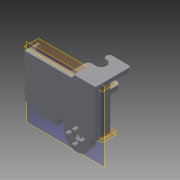
# Autodesk Inventor part: servo-holder
Saved by Autodesk Inventor 2014 (Build 180170000, 170)
## iProperties
Created: 2015-03-09
Part Number: servo-holder
Material: 一般
Document SubType Name: Modeling
Designer: Hideyuki Takei
Density: 1 g/cm^3
Appearance: 既定
d0: 14.000 mm
d1: 1.000 mm
d2: 0.00 deg
d3: 3.800 mm
d4: 8.800 mm
d5: 35.800 mm
d6: 22.000 mm
d7: 1.000 mm
d8: 1.000 mm
d9: 22.000 mm
d10: 22.000 mm
d11: 6.000 mm
d12: 0.00 deg
d14: 1.000 mm
d15: 22.000 mm
d16: 35.800 mm
d17: 8.800 mm
d18: 3.800 mm
d20: 0.00 deg
d23: 5.100 mm
d24: 3.100 mm
d25: 3.800 mm
d27: 5.600 mm
d28: 6.200 mm
d29: 2.100 mm
d30: 2.100 mm
d31: 3.600 mm
d32: 24.900 mm
d33: 5.500 mm
d34: 8.000 mm
d35: 0.000 mm
d36: 0.000 mm
d37: 5.300 mm
d38: 0.000 mm
d39: 0.000 mm
d40: 8.000 mm
d41: 1.000 mm
d42: 0.00 deg
d43: 22.000 mm
d54: 0.000 mm
d55: 0.000 mm
d56: 11.500 mm
d57: 19.000 mm
d58: 5.800 mm
d59: 9.800 mm
d60: 12.800 mm
d61: 5.800 mm
d62: 2.900 mm
d63: 5.740 mm
d64: 2.000 mm
d65: 0.00 deg
d66: 5.800 mm
d67: 9.900 mm
d68: 0.000 mm
d69: 9.138 mm
d70: 2.000 mm
d71: 0.00 deg
d72: 3.000 mm
d73: 1.200 mm
d74: 2.000 mm
d75: 2.000 mm
d76: 3.100 mm
d78: 0.00 deg
d79: -1.500 mm
d80: 0.000 mm
d81: 0.000 mm
d82: 34.000 mm
d83: 12.000 mm
d84: 2.300 mm
d85: 0.00 deg
d86: 3.000 mm
d87: 12.000 mm
d88: 0.000 mm
d89: 0.000 mm
d91: 0.00 deg
d93: 0.000 mm
d94: 0.000 mm
d95: 0.000 mm
d96: 1.000 mm
d97: 0.00 deg
d98: 0.500 mm
d99: 2.800 mm
d100: 0.00 deg
d101: 19.000 mm
d103: 3.600 mm
d104: 2.500 mm
d105: 0.00 deg
d106: 2.000 mm
d108: 5.300 mm
d109: 1.500 mm
d111: 1.500 mm
d112: 5.000 mm
d113: 2.000 mm
d114: 0.00 deg
d115: 1.500 mm
d116: 3.200 mm
d117: 10.800 mm
d118: 16.000 mm
d119: 17.000 mm
d121: 0.00 deg
d122: 10.000 mm
d123: 0.500 mm
d124: 0.00 deg
d125: 5.000 mm
d126: 3.200 mm
d127: 3.700 mm
d128: 0.00 deg
d131: 1.000 mm
d132: 0.00 deg
d134: 2.000 mm
d135: 0.00 deg
d136: 5.600 mm
d137: 1.800 mm
d138: 0.00 deg
d139: 2.000 mm
d140: 0.00 deg
d141: 5.500 mm
d142: 7.000 mm
d143: 2.500 mm
d144: 3.500 mm
d145: 3.500 mm
d146: 3.500 mm
d147: 3.500 mm
d148: 2.500 mm
d149: 2.500 mm
d150: 2.500 mm
d151: 2.000 mm
d152: 0.00 deg
d153: 0.500 mm
Author: Hideyuki Takei
Autodesk Inventor part; units mm, degrees
ref_plane "YZ Plane" through (0, 0, 0) normal (1, 0, 0) x (0, 1, 0)
sketch "スケッチ2" plane through (0, 0, 0) normal (0, 1, 0) x (-1, 0, 0)
  line L0 (-8.8, 25.8) -> (27, 25.8)
  line L1 (27, 25.8) -> (27, 3.8)
  line L2 (27, 3.8) -> (-8.8, 3.8)
  line L3 (-8.8, 3.8) -> (-8.8, 25.8)
  line L4 (-8.8, 25.8) -> (-9.8, 25.8)
  line L5 (-9.8, 25.8) -> (-9.8, 3.8)
  line L6 (-9.8, 3.8) -> (-8.8, 3.8)
  line L7 (-8.8, 3.8) -> (-8.8, 25.8)
  line L8 (27, 25.8) -> (28, 25.8)
  line L9 (28, 25.8) -> (28, 3.8)
  line L10 (28, 3.8) -> (27, 3.8)
  line L11 (27, 3.8) -> (27, 25.8)
  point P0 (0, 0)
  dimension "d3" = 3.8
  dimension "d4" = 8.8
  dimension "d5" = 35.8
  dimension "d6" = 22
  dimension "d7" = 1
  dimension "d8" = 1
  dimension "d9" = 22
  dimension "d10" = 22
  constraints: 24 end point, 6 parallel, 3 horizontal, 3 perpendicular
  measures "d3" distance from line of point (0, 0) L2
  measures "d4" distance from line of point (0, 0) L3
  measures "d5" distance of L0.start L0.end
  measures "d6" distance of L2.end L0.start
  measures "d7" distance of L0.start L4.end
  measures "d8" distance of L0.end L8.end
  measures "d9" distance of L8.end L9.end
  measures "d10" distance of L4.end L5.end
extrude "押し出し2" add sketch "スケッチ2" along normal blind 6 and the other way blind 2
ref_plane "作業平面4" through (0, 1, 0) normal (0, 1, 0) x (-1, 0, 0)
sketch "スケッチ3" plane through (0, 1, 0) normal (0, 1, 0) x (-1, 0, 0)
  line L0 (-8.8, 3.8) -> (27, 3.8)
  line L1 (27, 3.8) -> (27, 25.8)
  line L2 (27, 25.8) -> (-8.8, 25.8)
  line L3 (-8.8, 25.8) -> (-8.8, 3.8)
  point P0 (0, 0)
  dimension "d15" = 22
  dimension "d16" = 35.8
  dimension "d17" = 8.8
  dimension "d18" = 3.8
  constraints: 8 end point, 2 parallel, 1 horizontal, 1 perpendicular
  measures "d15" distance of L2.end L0.start
  measures "d16" distance of L1.end L2.end
  measures "d17" distance from line of point (0, 0) L3
  measures "d18" distance from line of point (0, 0) L0
extrude "押し出し3" cut sketch "スケッチ3" along normal up to next
fillet "フィレット3" radius 5.1 1 edges at (8.8, 1, 14.8)
sketch "スケッチ1" plane through (0, 0, 0) normal (0, 1, 0) x (-1, 0, 0)
  circle A0 centre (0, 0) radius 7
  dimension "d0" = 14
  constraints: 1 centre point, 1 coincident
  measures "d0" diameter of A0
extrude "押し出し1" add sketch "スケッチ1" along normal blind 1 and the other way blind 2
fillet "フィレット4" radius 3.1 1 edges at (-27, 1, 14.8)
ref_plane "作業平面5" through (0, 0, 3.8) normal (0, 0, 1) x (1, 0, 0)
sketch "スケッチ4" plane through (0, 0, 3.8) normal (0, 0, 1) x (1, 0, 0)
  circle A0 centre (6.2, 3.6) radius 1.05
  line L0 (-7, -2) -> (7, -2) projected
  circle A1 centre (-24.9, 3.6) radius 1.05
  line L1 (9.8, 6) -> (4.3, 6)
  line L2 (4.3, 6) -> (4.3, -2)
  line L3 (4.3, -2) -> (9.8, -2)
  line L4 (9.8, -2) -> (9.8, 6)
  line L5 (9.8, -2) -> (9.8, 6) projected
  line L6 (-28, 6) -> (-22.7, 6)
  line L7 (-22.7, 6) -> (-22.7, -2)
  line L8 (-22.7, -2) -> (-28, -2)
  line L9 (-28, -2) -> (-28, 6)
  line L10 (-28, -2) -> (-28, 6) projected
  line L11 (-28, -2) -> (-5.8788, -2) projected
  point P0 (0, 0)
  point P1 (5.8788, -2)
  dimension "d27" = 5.6
  dimension "d28" = 6.2
  dimension "d29" = 2.1
  dimension "d30" = 2.1
  dimension "d31" = 3.6
  dimension "d32" = 24.9
  dimension "d33" = 5.5
  dimension "d34" = 8
  dimension "d35" = 0
  dimension "d36" = 0
  dimension "d37" = 5.3
  dimension "d38" = 0
  dimension "d39" = 0
  dimension "d40" = 8
  constraints: 16 end point, 4 parallel, 2 centre point, 2 horizontal, 2 perpendicular, 1 other
  measures "d28" horizontal distance of point (0, 0) A0.centre
  measures "d29" diameter of A0
  measures "d30" diameter of A1
  measures "d31" vertical distance of point (0, 0) A1.centre
  measures "d32" horizontal distance of A1.centre point (0, 0)
  measures "d33" distance of L1.start L1.end
  measures "d34" distance of L1.end L2.end
  measures "d35" vertical extent of L3
  measures "d36" distance between parallel lines of L5 L4
  measures "d37" distance of L6.start L6.end
  measures "d38" distance between parallel lines of L10 L9
  measures "d39" distance between parallel lines of L11 L8
  measures "d40" distance of L6.end L7.end
extrude "押し出し4" add sketch "スケッチ4" against normal blind 1
ref_plane "作業平面7" through (0, 0, 25.8) normal (0, 0, 1) x (1, 0, 0)
sketch "スケッチ6" plane through (0, 0, 25.8) normal (0, 0, 1) x (1, 0, 0)
  line L0 (9.8, -2) -> (-1.7, -2)
  line L1 (-1.7, -2) -> (-1.7, 17)
  line L2 (-1.7, 17) -> (9.8, 17)
  line L3 (9.8, 17) -> (9.8, -2)
  line L4 (9.8, -2) -> (9.8, 6) projected
  line L5 (9.8, -2) -> (-28, -2) projected
  circle A0 centre (0, 10.8) radius 2.9
  line L6 (0, 13.7) -> (-5.7401, 13.7)
  line L7 (-5.7401, 13.7) -> (-5.7401, 7.9)
  line L8 (-5.7401, 7.9) -> (0, 7.9)
  line L9 (0, 7.9) -> (0, 13.7)
  line L10 (9.8, 16.7501) -> (9.8, 6)
  point P0 (0, 0)
  point P1 (-28, -2)
  dimension "d58" = 5.8
  dimension "d54" = 0
  dimension "d55" = 0
  dimension "d56" = 11.5
  dimension "d57" = 19
  dimension "d59" = 9.8
  dimension "d60" = 12.8
  dimension "d61" = 5.8
  dimension "d62" = 2.9
  dimension "d63" = 5.7401
  constraints: 18 end point, 4 parallel, 2 horizontal, 2 perpendicular, 1 point on line, 1 vertical alignment, 3 other
  measures "d54" distance between parallel lines of L4 L3
  measures "d55" vertical extent of L0
  measures "d56" distance of L1.end L2.end
  measures "d57" distance of L2.end L0.start
  measures "d59" distance from line of L3 point (0, 10.8)
  measures "d60" distance from line of L0 point (0, 10.8)
  measures "d61" distance of L6.end L7.end
  measures "d62" distance from line of L8 point (0, 10.8)
  measures "d63" distance of L6.start L6.end
extrude "押し出し5" add sketch "スケッチ6" along normal blind 2 contours L0 L1 L8 A0 L6 L2 L3 | L1 A0 L8 | L1 L6 A0
sketch "スケッチ7" plane through (0, 0, 25.8) normal (0, 0, 1) x (1, 0, 0)
  line L0 (0, 13.7) -> (-9.1376, 13.7)
  line L1 (-9.1376, 13.7) -> (-9.1376, 7.9)
  line L2 (-9.1376, 7.9) -> (0, 7.9)
  line L3 (0, 7.9) -> (0, 13.7)
  line L4 (-1.7, -2) -> (9.8, -2) projected
  point P0 (0, 0)
  dimension "d66" = 5.8
  dimension "d67" = 9.9
  dimension "d68" = 0
  dimension "d69" = 9.1376
  constraints: 8 end point, 2 parallel, 1 horizontal, 1 perpendicular, 1 other
  measures "d66" distance of L0.end L1.end
  measures "d68" distance from line of point (0, 0) L3
  measures "d69" distance of L0.start L0.end
extrude "押し出し6" cut sketch "スケッチ7" along normal blind 2
fillet "フィレット5" radius 3 1 edges at (4.3, 6, 3.3)
fillet "フィレット6" radius 1.2 5 edges at (-1.7, 17, 26.8) (-1.7, 13.7, 26.8) (9.8, 17, 26.8) (-1.7, 7.9, 26.8) (-27.5, 6, 25.8)
fillet "フィレット7" radius 2 1 edges at (-1.7, -0.5, 25.8)
fillet "フィレット8" radius 2 3 edges at (4.3, 1, 3.3) (-5.8788, -0.5, 3.8) (6.4156, -0.5, 2.8)
sketch "スケッチ8" plane through (0, 1, 0) normal (0, 1, 0) x (-1, 0, 0)
  circle A0 centre (0, 0) radius 1.55
  dimension "d76" = 3.1
  constraints: 1 centre point, 1 coincident
  measures "d76" diameter of A0
extrude "押し出し7" cut sketch "スケッチ8" against normal up to next
ref_plane "作業平面8" through (0, 0, 2.3) normal (0, 0, 1) x (1, 0, 0)
sketch "スケッチ9" plane through (0, 0, 2.3) normal (0, 0, 1) x (1, 0, 0)
  line L0 (-10.7, 32) -> (-22.7, 32)
  line L1 (-22.7, 32) -> (-22.7, -2)
  line L2 (-22.7, -2) -> (-10.7, -2)
  line L3 (-10.7, -2) -> (-10.7, 32)
  line L4 (-22.7, -2) -> (-5.8788, -2) projected
  line L5 (-22.7, 6) -> (-22.7, -2) projected
  point P0 (0, 0)
  point P1 (-8.8182, -2)
  dimension "d80" = 0
  dimension "d81" = 0
  dimension "d82" = 34
  dimension "d83" = 12
  constraints: 8 end point, 2 parallel, 1 horizontal, 1 perpendicular
  measures "d80" distance between parallel lines of L4 L2
  measures "d81" distance between parallel lines of L5 L1
  measures "d82" distance of L2.end L0.start
  measures "d83" distance of L0.start L0.end
extrude "押し出し8" add sketch "スケッチ9" against normal blind 2.3
sketch "スケッチ10" plane through (0, 0, 2.3) normal (0, 0, 1) x (1, 0, 0)
  line L0 (-10.7, 1) -> (-22.7, 1)
  line L1 (-22.7, 1) -> (-22.7, -2)
  line L2 (-22.7, -2) -> (-10.7, -2)
  line L3 (-10.7, -2) -> (-10.7, 1)
  line L4 (-10.7, 32) -> (-10.7, -2) projected
  line L5 (-10.7, -2) -> (-22.7, -2) projected
  point P0 (0, 0)
  dimension "d86" = 3
  dimension "d87" = 12
  dimension "d88" = 0
  dimension "d89" = 0
  constraints: 8 end point, 2 parallel, 1 horizontal, 1 perpendicular
  measures "d86" distance of L2.end L0.start
  measures "d87" distance of L1.end L2.end
  measures "d88" distance between parallel lines of L4 L3
  measures "d89" distance between parallel lines of L5 L2
extrude "押し出し9" add sketch "スケッチ10" along normal up to next
sketch "スケッチ11" plane through (0, 0, 3.8) normal (0, 0, 1) x (1, 0, 0)
  line L0 (-22.7, 32) -> (-28, 32)
  line L1 (-28, 32) -> (-28, 6)
  line L2 (-28, 6) -> (-22.7, 6)
  line L3 (-22.7, 6) -> (-22.7, 32)
  line L4 (-22.7, 1) -> (-22.7, -2) projected
  line L5 (-28, -2) -> (-28, 6) projected
  line L6 (-28, 6) -> (-22.7, 6) projected
  line L7 (-22.7, 32) -> (-10.7, 32) projected
  point P0 (0, 0)
  dimension "d93" = 0
  dimension "d94" = 0
  dimension "d95" = 0
  dimension "d108" = 5.3
  constraints: 8 end point, 2 parallel, 1 horizontal, 1 perpendicular
  measures "d93" distance between parallel lines of L5 L1
  measures "d94" distance between parallel lines of L6 L2
  measures "d95" distance between parallel lines of L7 L0
  measures "d108" distance between parallel lines of L1 L3
extrude "押し出し10" add sketch "スケッチ11" against normal blind 1
sketch "スケッチ12" plane through (0, 0, 2.8) normal (0, 0, -1) x (-1, 0, 0)
  line L0 (22.7, 32) -> (22.7, -2) projected
  line L1 (22.7, 1) -> (22.7, -2) projected
  line L2 (22.7, -2) -> (28, -2) projected
  line L3 (22.7, 32) -> (23.2, 32)
  line L4 (23.2, 32) -> (23.2, -2)
  line L5 (23.2, -2) -> (22.7, -2)
  line L6 (22.7, -2) -> (22.7, 32)
  point P0 (0, 0)
  dimension "d98" = 0.5
  constraints: 8 end point, 2 parallel, 1 horizontal, 1 perpendicular, 1 point on line
  measures "d98" distance of L0.start L3.end
extrude "押し出し11" add sketch "スケッチ12" along normal blind 2.8
fillet "フィレット13" radius 1.5 2 edges at (-23.2, 15, 0) (-23.2, 15, 2.8)
fillet "フィレット9" radius 19 1 edges at (-27.5, 6, 3.8)
sketch "スケッチ13" plane through (0, 0, 2.8) normal (0, 0, -1) x (-1, 0, 0)
  arc A0 (23.85, 3.6) -> (23.85, 3.6) centre (24.9, 3.6) ccw projected
  circle A1 centre (24.9, 3.6) radius 1.8
  point P0 (0, 0)
  dimension "d103" = 3.6
  constraints: 1 centre point, 1 coincident
  measures "d103" diameter of A1
extrude "押し出し12" cut sketch "スケッチ13" along normal blind 2.5 contours A0 | A1
fillet "フィレット11" radius 2 2 edges at (-28, 32, 3.3) (-10.7, 32, 1.15)
fillet "フィレット15" radius 1.5 1 edges at (-10.7, -0.5, 3.8)
sketch "スケッチ14" plane through (-22.7, 1, 2.3) normal (1, 0, 0) x (0, 0, -1)
  line L0 (0, 31) -> (0, 0) projected
  line L1 (-1.5, 31) -> (0, 31)
  line L2 (0, 31) -> (0, 26)
  line L3 (0, 26) -> (-1.5, 26)
  line L4 (-1.5, 26) -> (-1.5, 31)
  point P0 (2.3, -1)
  dimension "d112" = 5
  constraints: 8 end point, 2 parallel, 1 horizontal, 1 perpendicular, 1 point on line
  measures "d112" distance of L3.end L1.start
extrude "押し出し13" add sketch "スケッチ14" along normal blind 2
fillet "フィレット16" radius 1.5 1 edges at (-20.7, 29.5, 3.8)
sketch "スケッチ16" plane through (0, 0, 2.3) normal (0, 0, 1) x (1, 0, 0)
  circle A0 centre (-16, 25.8) radius 1.6
  line L0 (-1.7, -2) -> (9.8, -2) projected
  point P0 (0, 0)
  point P1 (0, 8.8)
  dimension "d116" = 3.2
  dimension "d117" = 10.8
  dimension "d118" = 16
  dimension "d119" = 17
  constraints: 1 centre point, 1 other
  measures "d116" diameter of A0
  measures "d118" horizontal distance of point (0, 8.8) A0.centre
  measures "d119" vertical distance of A0.centre point (0, 8.8)
extrude "押し出し14" cut sketch "スケッチ16" against normal up to next
sketch "スケッチ17" plane through (0, 0, 0) normal (0, 0, -1) x (-1, 0, 0)
  circle A0 centre (16, 25.8) radius 1.6 projected
  circle A1 centre (16, 25.8) radius 5
  point P0 (0, 0)
  dimension "d122" = 10
  constraints: 1 centre point, 1 coincident
  measures "d122" diameter of A1
extrude "押し出し15" add sketch "スケッチ17" along normal blind 0.5
sketch "スケッチ18" plane through (0, 0, 0) normal (0, 0, -1) x (-1, 0, 0)
  circle A0 centre (16, 25.8) radius 5 projected
  circle A1 centre (16, 25.8) radius 1.6
  circle A2 centre (16, 25.8) radius 2.5
  point P0 (0, 0)
  dimension "d125" = 5
  dimension "d126" = 3.2
  constraints: 2 centre point, 2 coincident
  measures "d125" diameter of A2
  measures "d126" diameter of A1
extrude "押し出し16" add sketch "スケッチ18" along normal blind 3.7 contours A2
sketch "スケッチ19" plane through (0, 0, 2.3) normal (0, 0, 1) x (1, 0, 0)
  circle A0 centre (-16, 25.8) radius 1.6 projected
  line L0 (-14.4239, 28.5567) -> (-12.8246, 25.8134)
  line L1 (-12.8246, 25.8134) -> (-14.4007, 23.0567)
  line L2 (-14.4007, 23.0567) -> (-17.5761, 23.0433)
  line L3 (-17.5761, 23.0433) -> (-19.1754, 25.7866)
  line L4 (-19.1754, 25.7866) -> (-17.5993, 28.5433)
  line L5 (-17.5993, 28.5433) -> (-14.4239, 28.5567)
  line L6 (-13.9765, 29.2984) -> (-11.9585, 25.7968)
  line L7 (-11.9585, 25.7968) -> (-13.982, 22.2984)
  line L8 (-13.982, 22.2984) -> (-18.0235, 22.3016)
  line L9 (-18.0235, 22.3016) -> (-20.0415, 25.8032)
  line L10 (-20.0415, 25.8032) -> (-18.018, 29.3016)
  line L11 (-18.018, 29.3016) -> (-13.9765, 29.2984)
  point P0 (0, 0)
  dimension "d141" = 5.5
  dimension "d142" = 7
  constraints: 24 end point, 2 coincident, 26 other
  measures "d141" distance between parallel lines of L2 L5
  measures "d142" distance between parallel lines of L8 L11
extrude "押し出し17" add sketch "スケッチ19" along normal blind 1 contours L6 L7 L8 L9 L10 L11
sketch "スケッチ21" plane through (0, 1, 0) normal (0, 1, 0) x (-1, 0, 0)
  line L0 (0, 3.2332) -> (2.8, 1.6166)
  line L1 (2.8, 1.6166) -> (2.8, -1.6166)
  line L2 (2.8, -1.6166) -> (0, -3.2332)
  line L3 (0, -3.2332) -> (-2.8, -1.6166)
  line L4 (-2.8, -1.6166) -> (-2.8, 1.6166)
  line L5 (-2.8, 1.6166) -> (0, 3.2332)
  point P0 (0, 0)
  point P1 (0, 0)
  dimension "d136" = 5.6
  constraints: 12 end point, 1 coincident, 13 other
  measures "d136" distance between parallel lines of L1 L4
extrude "押し出し18" cut sketch "スケッチ21" against normal blind 1.8
sketch "スケッチ22" plane through (0, -2, 0) normal (0, -1, 0) x (1, 0, 0)
  arc A0 (-6.8586, 1.4) -> (6.9723, 0.6222) centre (0, 0) ccw projected
  circle A1 centre (0, 0) radius 1.55 projected
  circle A2 centre (-3.5, 0) radius 1.25
  circle A3 centre (0, 3.5) radius 1.25
  circle A4 centre (3.5, 0) radius 1.25
  circle A5 centre (0, -3.5) radius 1.25
  dimension "d143" = 2.5
  dimension "d144" = 3.5
  dimension "d145" = 3.5
  dimension "d146" = 3.5
  dimension "d147" = 3.5
  dimension "d148" = 2.5
  dimension "d149" = 2.5
  dimension "d150" = 2.5
  constraints: 4 centre point
  measures "d143" diameter of A2
  measures "d144" distance of A0.centre A2.centre
  measures "d145" distance of A0.centre A3.centre
  measures "d146" distance of A4.centre A1.centre
  measures "d147" distance of A0.centre A5.centre
  measures "d148" diameter of A3
  measures "d149" diameter of A4
  measures "d150" diameter of A5
extrude "押し出し19" add sketch "スケッチ22" along normal blind 2 contours A2 | A3 | A4 | A5
fillet "フィレット17" radius 0.5 4 edges at (-1.25, -4, -3.5) (-4.75, -4, 0) (-1.25, -4, 3.5) (2.25, -4, 0)
equation "\"d30\" = d29"
equation "\"d62\" = 0.5 * d61"
